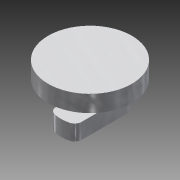
# Autodesk Inventor part: EarConnector
Saved by Autodesk Inventor 2014 SP1 (Build 180222100, 222)
## iProperties
Created: 2013-10-30
Part Number: EarConnector
Material: Generic
Document SubType Name: Modeling
Designer: david
Density: 1 g/cm^3
Appearance: Machined - Aluminum
EarConnectorHeight: 3,000 mm
Author: david
Autodesk Inventor part; units mm, degrees
ref_plane "YZ Plane" through (0, 0, 0) normal (1, 0, 0) x (0, 1, 0)
ref_plane "XZ Plane" through (0, 0, 0) normal (0, 1, 0) x (-1, 0, 0)
ref_plane "XY Plane" through (0, 0, 0) normal (0, 0, 1) x (1, 0, 0)
sketch "Sketch1" plane through (0, 0, 0) normal (0, 1, 0) x (-1, 0, 0)
  circle A0 centre (0, 0) radius 7.5
  dimension "d0" = 15
  constraints: 1 centre point, 1 coincident
  measures "d0" diameter of A0
extrude "Extrusion1" add sketch "Sketch1" along normal blind 3
sketch "Sketch2" plane through (0, 0, 0) normal (0, -1, 0) x (1, 0, 0)
  circle A0 centre (0, 0) radius 7.5 projected
  circle A1 centre (0, 0) radius 2.3
  dimension "d3" = 4.6
  constraints: 1 centre point, 1 coincident
  measures "d3" diameter of A1
extrude "Extrusion2" add sketch "Sketch2" along normal blind 3.6 contours A1
sketch "Sketch3" plane through (0, -3.6, 0) normal (0, -1, 0) x (1, 0, 0)
  circle A0 centre (0, 0) radius 2.3 projected
  line L0 (-2.3, 4.6637) -> (-2.3, -5.1059)
  line L1 (2.3, 4.6637) -> (2.3, -5.1059)
  line L2 (0, 15.7328) -> (0, -15.032) construction
  circle A1 centre (0, 0) radius 7.5 construction
  arc A2 (-3, 6.8739) -> (-3, -6.8739) centre (0, 0) ccw construction
  arc A3 (3, -6.8739) -> (3, 6.8739) centre (0, 0) ccw construction
  arc A4 (2.3, 4.6637) -> (-2.3, 4.6637) centre (0, 0) ccw
  arc A5 (-2.3, -5.1059) -> (2.3, -5.1059) centre (0, 0) ccw
  dimension "d13" = 5.2
  dimension "d19" = 5.6
  constraints: 12 point on circle, 6 end point, 4 centre point, 2 coincident, 2 parallel, 2 tangent, 1 concentric, 1 vertical
  measures "d13" radius of A4
  measures "d19" radius of A5
extrude "Extrusion3" add sketch "Sketch3" along normal blind 2.8
fillet "Fillet2" radius 1.2 4 edges at (-2.3, -5, 4.6637) (2.3, -5, 4.6637) (-2.3, -5, -5.1059) (2.3, -5, -5.1059)
equation "\"d0\" = HeadConnectorOuterSize"
equation "\"d1\" = EarConnectorHeight"
equation "\"d3\" = HeadConnectorWidth - HeadConnectorTolerance"
equation "\"d4\" = HeadConnectorOuterHeight + 3 * HeadConnectorTolerance"
equation "\"d13\" = 0.5 * HeadConnectorDiam - 4 * HeadConnectorTolerance"
equation "\"d19\" = 0.5 * HeadConnectorDiam - 2 * HeadConnectorTolerance"
equation "\"d10\" = HeadConnectorHeight - HeadConnectorTolerance"
equation "\"d20\" = 2 * HeadConnectorProportion"
equation "\"EarConnectorHeight\" = 5 * HeadConnectorProportion"
equation "\"HeadConnectorOuterSize\" = 15"
equation "\"HeadConnectorWidth\" = 4.8"
equation "\"HeadConnectorTolerance\" = 0.2"
equation "\"HeadConnectorOuterHeight\" = 3"
equation "\"HeadConnectorDiam\" = 12"
equation "\"HeadConnectorHeight\" = 3"
equation "\"HeadConnectorProportion\" = 0.6"
body "Solid1"
